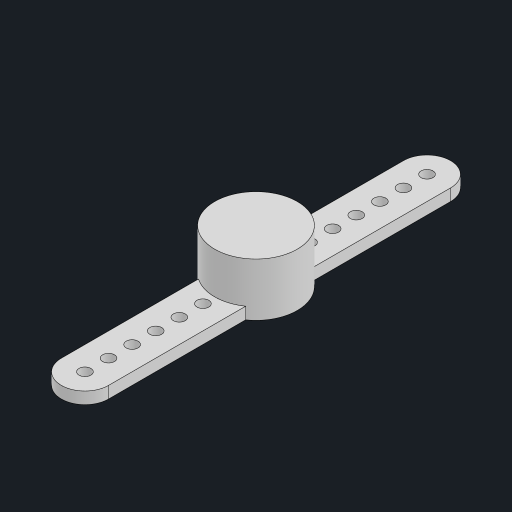
# Autodesk Inventor part: horn_10g
Saved by Autodesk Inventor 2023 (Build 270158000, 158)
## iProperties
Created: 2022-06-07
Part Number: horn_10g
Material: Generic
Document SubType Name: Modeling
Designer: legot
Density: 1 g/cm^3
Appearance: Default
Author: legot
Autodesk Inventor part; units mm, degrees
ref_plane "YZ Plane" through (0, 0, 0) normal (1, 0, 0) x (0, 1, 0)
ref_plane "XZ Plane" through (0, 0, 0) normal (0, 1, 0) x (-1, 0, 0)
ref_plane "XY Plane" through (0, 0, 0) normal (0, 0, 1) x (1, 0, 0)
sketch "スケッチ1" plane through (0, 0, 0) normal (0, 1, 0) x (-1, 0, 0)
  circle A0 centre (0, 0) radius 3.5
  circle A1 centre (0, 14.5) radius 2
  circle A2 centre (0, -14.5) radius 2
  line L0 (2, 14.5) -> (2, 2.8723)
  line L1 (-2, 14.5) -> (-2, 2.8723)
  line L2 (-2, -2.8723) -> (-2, -14.5)
  line L3 (2, -2.8723) -> (2, -14.5)
  dimension "d0" = 7
  dimension "d2" = 4
  dimension "d3" = 14.5
  dimension "d4" = 14.5
  constraints: 8 end point, 8 point on circle, 4 tangent, 4 vertical, 3 centre point, 2 vertical alignment, 1 coincident, 1 equal radius
  measures "d0" diameter of A0
  measures "d2" diameter of A2
  measures "d3" distance of point (0, 0) A1.centre
  measures "d4" distance of A2.centre point (0, 0)
extrude "押し出し1" add sketch "スケッチ1" along normal blind 1
sketch "スケッチ2" plane through (0, 1, 0) normal (0, 1, 0) x (1, 0, 0)
  arc A0 (-2, 2.8723) -> (-2, -2.8723) centre (0, 0) ccw projected
  circle A1 centre (0, 0) radius 3.5 projected
extrude "押し出し2" add sketch "スケッチ2" along normal blind 3.5
sketch "スケッチ3" plane through (0, 0, 0) normal (0, -1, 0) x (1, 0, 0)
  arc A0 (2, 14.5) -> (-2, 14.5) centre (0, 14.5) ccw projected
  point P0 (0, 12.5)
  point P1 (0, 10.5)
  point P2 (0, 8.5)
  point P3 (0, 6.5)
  point P4 (0, 4.5)
  dimension "d9" = 2
  dimension "d18" = 2
  dimension "d19" = 2
  dimension "d20" = 2
  dimension "d21" = 2
  constraints: 5 vertical alignment, 1 coincident
  measures "d9" distance of point (0, 12.5) point (0, 14.5)
  measures "d18" distance of point (0, 10.5) point (0, 12.5)
  measures "d19" distance of point (0, 10.5) point (0, 8.5)
  measures "d20" distance of point (0, 8.5) point (0, 6.5)
  measures "d21" distance of point (0, 6.5) point (0, 4.5)
hole "穴1" at (0, 0, 14.5) at (0, 0, 12.5) at (0, 0, 10.5) at (0, 0, 8.5) at (0, 0, 6.5) at (0, 0, 4.5) direction (0, 1, 0) diameter 1 end through all
mirror "ミラー1" about plane through (0, 0, 0) normal (0, 0, 1) of "穴1"
equation "\"d4\" = d3"
equation "\"d18\" = d9"
equation "\"d19\" = d9"
equation "\"d20\" = d9"
equation "\"d21\" = d9"
